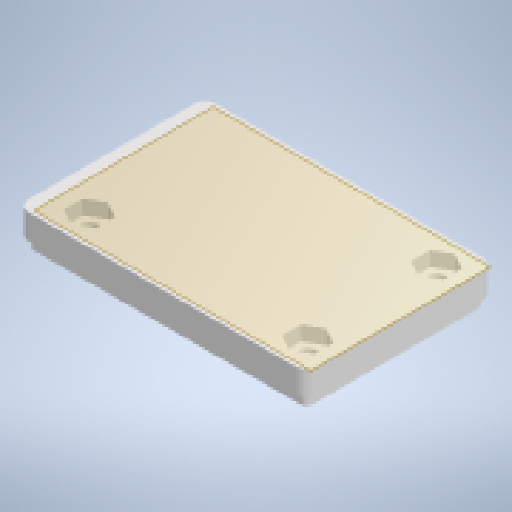
# Autodesk Inventor part: Gehaeuse_unten
Saved by Autodesk Inventor 2024 (Build 280153000, 153)
## iProperties
Created: 2025-04-09
Part Number: Gehaeuse_unten
Material: Generisch
Document SubType Name: Modeling
Designer: erikt
Density: 1 g/cm^3
Appearance: Vorgabe
Author: erikt
Autodesk Inventor part; units mm, degrees
ref_plane "YZ Plane" through (0, 0, 0) normal (1, 0, 0) x (0, 1, 0)
ref_plane "XZ Plane" through (0, 0, 0) normal (0, 1, 0) x (-1, 0, 0)
ref_plane "XY Plane" through (0, 0, 0) normal (0, 0, 1) x (1, 0, 0)
ref_plane "Arbeitsebene1" through (0, 0, 6) normal (0, 0, 1) x (1, 0, 0)
sketch "Skizze3" plane through (0, 0, 6) normal (0, 0, 1) x (1, 0, 0)
  line L0 (22.5, -14.565) -> (22.5, 14.565) projected
  line L1 (-22.5, -14.565) -> (22.5, -14.565) projected
  line L2 (-22.5, 14.565) -> (-22.5, -14.565) projected
  line L3 (22.5, 14.565) -> (-22.5, 14.565) projected
  circle A0 centre (19.6, -11.465) radius 1.5 projected
  circle A1 centre (13.06, -2.125) radius 0.65 projected
  circle A2 centre (13.06, -4.665) radius 0.65 projected
  circle A3 centre (13.06, 0.415) radius 0.65 projected
  circle A4 centre (13.06, 2.955) radius 0.65 projected
  circle A5 centre (-2.18, 5.495) radius 0.65 projected
  circle A6 centre (13.06, 5.495) radius 0.65 projected
  circle A7 centre (19.6, 11.535) radius 1.5 projected
  circle A8 centre (13.06, 8.035) radius 0.65 projected
  circle A9 centre (13.06, 10.575) radius 0.65 projected
  circle A10 centre (-2.18, 8.035) radius 0.65 projected
  circle A11 centre (13.06, 13.115) radius 0.65 projected
  circle A12 centre (-2.18, 10.575) radius 0.65 projected
  circle A13 centre (-7.26, -6.945) radius 0.5 projected
  circle A14 centre (-2.18, -2.125) radius 0.65 projected
  circle A15 centre (-2.18, -4.665) radius 0.65 projected
  circle A16 centre (-12.34, -6.945) radius 0.5 projected
  circle A17 centre (-19.4, -11.465) radius 1.5 projected
  circle A18 centre (-7.26, -4.405) radius 0.5 projected
  circle A19 centre (-12.34, -4.405) radius 0.5 projected
  circle A20 centre (-2.18, 0.415) radius 0.65 projected
  circle A21 centre (-2.18, 13.115) radius 0.65 projected
  circle A22 centre (-2.18, 2.955) radius 0.65 projected
  circle A23 centre (-7.26, -1.865) radius 0.5 projected
  circle A24 centre (-12.34, -1.865) radius 0.5 projected
  circle A25 centre (-7.26, 0.675) radius 0.5 projected
  circle A26 centre (-12.34, 0.675) radius 0.5 projected
  line L4 (-24.7, -16.765) -> (24.7, -16.765)
  line L5 (24.7, -16.765) -> (24.7, 16.765)
  line L6 (24.7, 16.765) -> (-24.7, 16.765)
  line L7 (-24.7, 16.765) -> (-24.7, -16.765)
  line L8 (-24.34, 2.175) -> (-10.84, 2.175) projected
  line L9 (-10.84, 2.175) -> (-10.84, -8.525) projected
  line L10 (-10.84, -8.525) -> (-24.34, -8.525) projected
  line L11 (-24.34, -8.525) -> (-24.34, 2.175) projected
  circle A27 centre (-12.34, -1.865) radius 0.5 projected
  circle A28 centre (-12.34, -4.405) radius 0.5 projected
  circle A29 centre (-12.34, -6.945) radius 0.5 projected
  circle A30 centre (-12.34, 0.675) radius 0.5 projected
  circle A31 centre (-21.39, -0.725) radius 1.5 projected
  line L12 (24.7, 16.765) -> (-26.94, 16.765)
  line L13 (-26.94, 16.765) -> (-26.94, -16.765)
  line L14 (-26.94, -16.765) -> (24.7, -16.765)
  line L15 (24.7, -16.765) -> (24.7, 16.765)
  point P0 (0, 0)
  point P1 (-24.7, 16.765)
  dimension "d5" = 2.2
  dimension "d6" = 2.6
  constraints: 16 end point, 2 parallel, 1 horizontal, 1 perpendicular, 3 other
  measures "d5" distance between parallel lines of L2 L7
  measures "d6" distance between parallel lines of L13 L11
extrude "Extrusion2" add sketch "Skizze3" against normal blind 2 contours L1 L2 L10 L9 L8 L3 L0 | L10 L11 L8 L2 A31 | L2 A31 L8 L9 L10 | A31 L2 | L2 A31 | A0 | A1 | A2 | A3 | A4 | A5 | A6 | A7 | A8 | A9 | A10 | A11 | A12 | A13 | A14 | A15 | A16 | A17 | A18 | A19 | A20 | A21 | A22 | A23 | A24 | A25 | A26 | L7 L6 L5 L4 | L14 L13 L12 L7
sketch "Skizze4" plane through (0, 0, 4) normal (0, 0, -1) x (-1, 0, 0)
  line L0 (-24.7, 16.765) -> (-24.7, -16.765) projected
  line L1 (-24.7, -16.765) -> (26.94, -16.765) projected
  line L2 (26.94, -16.765) -> (26.94, 16.765) projected
  line L3 (26.94, 16.765) -> (-24.7, 16.765) projected
  line L4 (-22.7, 14.765) -> (-22.7, -14.765)
  line L5 (-22.7, -14.765) -> (24.94, -14.765)
  line L6 (24.94, -14.765) -> (24.94, 14.765)
  line L7 (24.94, 14.765) -> (-22.7, 14.765)
  point P0 (0, 0)
  dimension "d9" = 2
  constraints: 8 end point, 3 other
  measures "d9" distance between parallel lines of L3 L7
ref_plane "Arbeitsebene2" through (-22.5, -14.565, -0.4115) normal (0, 0, -1) x (0, 1, 0)
extrude "Extrusion3" add sketch "Skizze4" along normal up to surface (4.4115 mm away)
sketch "Skizze5" plane through (24.7, -16.765, -0.4115) normal (0, 0, -1) x (-1, 0, 0)
  line L0 (2, 31.53) -> (2, 2) projected
  line L1 (49.64, 31.53) -> (2, 31.53) projected
  line L2 (49.64, 2) -> (49.64, 31.53) projected
  line L3 (2, 2) -> (49.64, 2) projected
  line L4 (0, 0) -> (0, 33.53) projected
  line L5 (51.64, 0) -> (0, 0) projected
  line L6 (51.64, 33.53) -> (51.64, 0) projected
  line L7 (0, 33.53) -> (51.64, 33.53) projected
  line L8 (50.64, 32.53) -> (50.64, 1)
  line L9 (50.64, 1) -> (1, 1)
  line L10 (1, 1) -> (1, 32.53)
  line L11 (1, 32.53) -> (50.64, 32.53)
  point P0 (24.7, 16.765)
  dimension "d12" = 1
  constraints: 8 end point, 3 other
  measures "d12" distance between parallel lines of L7 L11
extrude "Extrusion4" cut sketch "Skizze5" against normal blind 2 contours L4 L7 L6 L5
sketch "Skizze6" plane through (0, 0, 4) normal (0, 0, -1) x (-1, 0, 0)
  circle A0 centre (-19.6, 11.535) radius 1.5 projected
  circle A1 centre (-19.6, -11.465) radius 1.5 projected
  circle A2 centre (19.4, -11.465) radius 1.5 projected
  circle A3 centre (-19.6, -11.465) radius 1.7
  circle A4 centre (-19.6, 11.535) radius 1.7
  circle A5 centre (19.4, -11.465) radius 1.7
  line L0 (-22.7, -14.765) -> (24.94, -14.765) projected
  line L1 (-22.7, -14.765) -> (-16.5, -14.765)
  line L2 (-16.5, -14.765) -> (-16.5, -10.165)
  line L3 (-18.5, -8.165) -> (-22.7, -8.165)
  line L4 (-22.7, -8.165) -> (-22.7, -14.765)
  arc A6 (-16.5, -10.165) -> (-18.5, -8.165) centre (-18.5, -10.165) ccw
  line L5 (24.94, 14.765) -> (-22.7, 14.765) projected
  line L6 (-22.7, 14.765) -> (-16.5, 14.765)
  line L7 (-16.5, 14.765) -> (-16.5, 10.165)
  line L8 (-18.5, 8.165) -> (-22.7, 8.165)
  line L9 (-22.7, 8.165) -> (-22.7, 14.765)
  line L10 (24.94, -14.765) -> (16.3, -14.765)
  line L11 (16.3, -14.765) -> (16.3, -10.165)
  line L12 (18.3, -8.165) -> (24.94, -8.165)
  line L13 (24.94, -8.165) -> (24.94, -14.765)
  arc A7 (18.3, -8.165) -> (16.3, -10.165) centre (18.3, -10.165) ccw
  arc A8 (-18.5, 8.165) -> (-16.5, 10.165) centre (-18.5, 10.165) ccw
  line L14 (24.94, 14.765) -> (16.3, 14.765)
  line L15 (16.3, 14.765) -> (16.3, 10.165)
  line L16 (18.3, 8.165) -> (24.94, 8.165)
  line L17 (24.94, 8.165) -> (24.94, 14.765)
  arc A9 (16.3, 10.165) -> (18.3, 8.165) centre (18.3, 10.165) ccw
  point P0 (0, 0)
  point P1 (-16.5, -8.165)
  point P2 (-16.5, 8.165)
  dimension "d15" = 0.2
  dimension "d16" = 0.2
  dimension "d17" = 0.2
  dimension "d18" = 6.2
  dimension "d19" = 6.6
  dimension "d20" = 2
  dimension "d21" = 6.2
  dimension "d22" = 6.6
  dimension "d23" = 3.3
  dimension "d24" = 3.1
  dimension "d25" = 2
  dimension "d26" = 2
  constraints: 32 end point, 8 parallel, 8 point on circle, 8 tangent, 7 centre point, 4 horizontal, 4 perpendicular, 4 point on line, 1 equal radius
  measures "d15" radial gap between concentric circles of A1 A3
  measures "d16" radial gap between concentric circles of A0 A4
  measures "d17" radial gap between concentric circles of A2 A5
  measures "d18" distance of L3.end point (-16.5, -8.165)
  measures "d19" distance of point (-16.5, -8.165) L1.end
  measures "d20" radius of A6
  measures "d21" distance of point (-16.5, 8.165) L8.end
  measures "d22" distance of L6.end point (-16.5, 8.165)
  measures "d23" distance from line of L12 A2.centre
  measures "d24" distance from line of L11 A2.centre
  measures "d25" radius of A7
  measures "d26" radius of A9
ref_plane "Arbeitsebene3" through (-22.5, -14.565, 0) normal (0, 0, 1) x (1, 0, 0)
extrude "Extrusion5" add sketch "Skizze6" along normal blind 2.211 contours L4 L3 A6 L2 L0 | L11 A7 L12 L13 L0 | L17 L16 A9 L15 L5 | L7 A8 L8 L9 L5
sketch "Skizze7" plane through (19.6, 11.535, 4) normal (0, 0, -1) x (-1, 0, 0)
  circle A0 centre (0, 0) radius 1.7 projected
  circle A1 centre (0, -23) radius 1.7 projected
  circle A2 centre (39, -23) radius 1.7 projected
  point P0 (19.6, -11.535)
extrude "Extrusion6" cut sketch "Skizze7" against normal up to surface (2 mm away)
sketch "Skizze8" plane through (0, 0, 6) normal (0, 0, 1) x (1, 0, 0)
  circle A0 centre (19.6, -11.465) radius 1.7 projected
  circle A1 centre (19.6, 11.535) radius 1.7 projected
  circle A2 centre (-19.4, -11.465) radius 1.7 projected
  line L0 (24.7, -16.765) -> (24.7, 16.765) projected
  line L1 (24.7, 16.765) -> (-26.94, 16.765) projected
  line L2 (-26.94, 16.765) -> (-26.94, -16.765) projected
  line L3 (-26.94, -16.765) -> (24.7, -16.765) projected
  line L4 (16.75, -9.8196) -> (19.6, -8.1741)
  line L5 (19.6, -8.1741) -> (22.45, -9.8196)
  line L6 (22.45, -9.8196) -> (22.45, -13.1104)
  line L7 (22.45, -13.1104) -> (19.6, -14.7559)
  line L8 (19.6, -14.7559) -> (16.75, -13.1104)
  line L9 (16.75, -13.1104) -> (16.75, -9.8196)
  line L10 (16.75, 13.1804) -> (19.6, 14.8259)
  line L11 (19.6, 14.8259) -> (22.45, 13.1804)
  line L12 (22.45, 13.1804) -> (22.45, 9.8896)
  line L13 (22.45, 9.8896) -> (19.6, 8.2441)
  line L14 (19.6, 8.2441) -> (16.75, 9.8896)
  line L15 (16.75, 9.8896) -> (16.75, 13.1804)
  line L16 (-22.25, -9.8196) -> (-19.4, -8.1741)
  line L17 (-19.4, -8.1741) -> (-16.55, -9.8196)
  line L18 (-16.55, -9.8196) -> (-16.55, -13.1104)
  line L19 (-16.55, -13.1104) -> (-19.4, -14.7559)
  line L20 (-19.4, -14.7559) -> (-22.25, -13.1104)
  line L21 (-22.25, -13.1104) -> (-22.25, -9.8196)
  line L22 (24.7, -16.765) -> (24.7, 16.765) projected
  point P0 (0, 0)
  dimension "d31" = 5.7
  dimension "d32" = 5.7
  dimension "d33" = 5.7
  constraints: 36 end point, 3 coincident, 3 parallel, 39 other
  measures "d31" distance between parallel lines of L9 L6
  measures "d32" distance between parallel lines of L21 L18
  measures "d33" distance between parallel lines of L15 L12
extrude "Extrusion7" cut sketch "Skizze8" against normal blind 2.6 contours A0 | A1 | A2 | L4 L5 L6 L7 L8 L9 | L10 L11 L12 L13 L14 L15 | L16 L17 L18 L19 L20 L21
fillet "Rundung1" radius 2 5 edges at (24.7, -16.765, 3.7943) (-26.94, -16.765, 3.7943) (-26.94, 16.765, 2.7943) (-26.94, 16.765, 5) (24.7, 16.765, 3.7943)
fillet "Rundung2" radius 1 4 edges at (-25.94, -15.765, 0.5885) (-25.94, 15.765, 0.5885) (23.7, 15.765, 0.5885) (23.7, -15.765, 0.5885)
